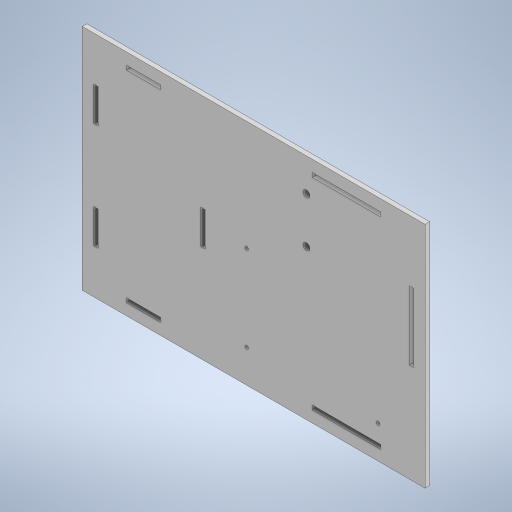
# Autodesk Inventor part: onderstuk_8AUG
Saved by Autodesk Inventor 2023.4 (Build 274418000, 418)
## iProperties
Created: 2024-07-29
Part Number: onderstuk_8AUG
Material: Generic
Document SubType Name: Modeling
Designer: cthey
Density: 1 g/cm^3
Appearance: Default
Author: cthey
Autodesk Inventor part; units mm, degrees
ref_plane "YZ Plane" through (0, 0, 0) normal (1, 0, 0) x (0, 1, 0)
ref_plane "XZ Plane" through (0, 0, 0) normal (0, 1, 0) x (-1, 0, 0)
ref_plane "XY Plane" through (0, 0, 0) normal (0, 0, 1) x (1, 0, 0)
sketch "Sketch1" plane through (0, 0, 0) normal (0, 0, 1) x (1, 0, 0)
  line L0 (0, 0) -> (300, 0)
  line L1 (300, 0) -> (300, 200)
  line L2 (300, 200) -> (0, 200)
  line L3 (0, 200) -> (0, 0)
  line L4 (10, 10) -> (290, 10)
  line L5 (290, 10) -> (290, 190)
  line L6 (290, 190) -> (10, 190)
  line L7 (10, 190) -> (10, 10)
  line L8 (13.75, 13.75) -> (286.25, 13.75)
  line L9 (286.25, 13.75) -> (286.25, 186.25)
  line L10 (286.25, 186.25) -> (13.75, 186.25)
  line L11 (13.75, 186.25) -> (13.75, 13.75)
  line L12 (38.75, 190) -> (68.5, 190)
  line L13 (68.5, 190) -> (68.5, 186.25)
  line L14 (68.5, 186.25) -> (38.75, 186.25)
  line L15 (38.75, 186.25) -> (38.75, 190)
  line L16 (10, 161.25) -> (13.75, 161.25)
  line L17 (13.75, 161.25) -> (13.75, 131.5)
  line L18 (13.75, 131.5) -> (10, 131.5)
  line L19 (10, 131.5) -> (10, 161.25)
  line L20 (0, 0) -> (150, 0)
  line L21 (150, 0) -> (150, 100)
  line L22 (150, 100) -> (0, 100)
  line L23 (0, 100) -> (0, 0)
  line L24 (38.75, 10) -> (68.5, 10)
  line L25 (68.5, 10) -> (68.5, 13.75)
  line L26 (68.5, 13.75) -> (38.75, 13.75)
  line L27 (38.75, 13.75) -> (38.75, 10)
  line L28 (10, 38.75) -> (13.75, 38.75)
  line L29 (13.75, 38.75) -> (13.75, 68.5)
  line L30 (13.75, 68.5) -> (10, 68.5)
  line L31 (10, 68.5) -> (10, 38.75)
  line L32 (150, 200) -> (150, 100)
  line L33 (300, 200) -> (300, 0)
  line L34 (261.25, 190) -> (231.5, 190)
  line L35 (231.5, 190) -> (231.5, 186.25)
  line L36 (231.5, 186.25) -> (261.25, 186.25)
  line L37 (261.25, 186.25) -> (261.25, 190)
  line L38 (290, 161.25) -> (286.25, 161.25)
  line L39 (286.25, 161.25) -> (286.25, 131.5)
  line L40 (286.25, 131.5) -> (290, 131.5)
  line L41 (290, 131.5) -> (290, 161.25)
  line L42 (300, 100) -> (300, 0)
  line L43 (261.25, 13.75) -> (261.25, 10)
  line L44 (231.5, 10) -> (231.5, 13.75)
  line L45 (231.5, 13.75) -> (261.25, 13.75)
  line L46 (261.25, 10) -> (231.5, 10)
  line L47 (286.25, 68.5) -> (290, 68.5)
  line L48 (290, 38.75) -> (286.25, 38.75)
  line L49 (290, 68.5) -> (290, 38.75)
  line L50 (286.25, 38.75) -> (286.25, 68.5)
  point P0 (13.75, 161.25)
  point P1 (10, 131.5)
  point P2 (10, 68.5)
  point P3 (13.75, 68.5)
  point P4 (13.75, 38.75)
  point P5 (10, 38.75)
  point P6 (68.5, 13.75)
  point P7 (68.5, 10)
  point P8 (38.75, 10)
  point P9 (38.75, 13.75)
  point P10 (231.5, 186.25)
  point P11 (231.5, 190)
  point P12 (261.25, 190)
  point P13 (261.25, 186.25)
  point P14 (286.25, 131.5)
  point P15 (286.25, 161.25)
  point P16 (290, 161.25)
  point P17 (261.25, 13.75)
  point P18 (261.25, 10)
  point P19 (231.5, 10)
  point P20 (231.5, 13.75)
  point P21 (286.25, 68.5)
  point P22 (286.25, 38.75)
  point P23 (68.5, 190)
  dimension "d0" = 300
  dimension "d1" = 200
  dimension "d2" = 280
  dimension "d3" = 180
  dimension "d4" = 10
  dimension "d5" = 10
  dimension "d6" = 3.75
  dimension "d7" = 3.75
  dimension "d8" = 3.75
  dimension "d9" = 3.75
  dimension "d10" = 25
  dimension "d11" = 29.75
  dimension "d12" = 29.75
  dimension "d13" = 25
  dimension "d14" = 100
  dimension "d15" = 150
  constraints: 102 end point, 26 symmetric about line, 12 parallel, 6 horizontal, 6 perpendicular, 4 point on line
  measures "d0" distance of L1.end L2.end
  measures "d1" distance of L0.end L1.end
  measures "d2" distance of L5.end L6.end
  measures "d3" distance of L6.end L4.start
  measures "d4" distance between parallel lines of L3 L7
  measures "d5" distance between parallel lines of L2 L6
  measures "d6" distance between parallel lines of L5 L9
  measures "d7" distance between parallel lines of L6 L10
  measures "d8" distance between parallel lines of L7 L11
  measures "d9" distance between parallel lines of L4 L8
  measures "d10" distance between parallel lines of L11 L15
  measures "d11" distance between parallel lines of L13 L15
  measures "d12" distance between parallel lines of L18 L16
  measures "d13" distance between parallel lines of L10 L16
  measures "d14" distance of L20.end L21.end
  measures "d15" distance of L21.end L22.end
extrude "Extrusion1" add sketch "Sketch1" along normal blind 4 contours L3 L22 L7 L4 L21 L0 | L21 L4 L5 L6 L32 L2 L1 L0 | L3 L2 L32 L6 L7 L22 | L21 L8 L44 L4 | L4 L25 L8 L21 | L22 L11 L30 L7 | L7 L18 L11 L22 | L21 L32 L10 L9 L8 | L8 L11 L22 L21 | L11 L10 L32 L22 | L4 L7 L28 L11 L8 L27 | L43 L8 L9 L48 L5 L4 | L32 L10 L13 L6 | L6 L35 L10 L32 | L7 L6 L15 L10 L11 L16 | L6 L5 L38 L9 L10 L37 | L47 L9 L40 L5
sketch "Sketch5" plane through (0, 0, 4) normal (0, 0, 1) x (1, 0, 0)
  line L0 (103.75, 114.875) -> (107.5, 114.875)
  line L1 (107.5, 114.875) -> (107.5, 85.125)
  line L2 (107.5, 85.125) -> (103.75, 85.125)
  line L3 (103.75, 85.125) -> (103.75, 114.875)
  line L4 (13.75, 68.5) -> (13.75, 38.75) projected
  line L5 (0, 0) -> (300, 0) projected
  point P0 (107.5, 100)
  dimension "d53" = 3.75
  dimension "d54" = 29.75
  dimension "d55" = 90
  dimension "d56" = 100
  constraints: 8 end point, 2 parallel, 1 horizontal, 1 midpoint, 1 perpendicular
  measures "d53" distance between parallel lines of L1 L3
  measures "d54" distance of L0.end L1.end
  measures "d55" distance between parallel lines of L4 L3
  measures "d56" distance from line of L5 point (107.5, 100)
extrude "Extrusion5" cut sketch "Sketch5" against normal through all
sketch "Sketch6" plane through (0, 0, 0) normal (0, 0, -1) x (-1, 0, 0)
  circle A0 centre (-258.8334, 28.75) radius 1.5
  circle A1 centre (-143.8334, 28.75) radius 1.5
  circle A2 centre (-143.8334, 103.75) radius 1.5
  line L0 (-300, 0) -> (-300, 200) projected
  line L1 (-231.5, 13.75) -> (-261.25, 13.75) projected
  circle A3 centre (-196.25, 171.25) radius 3
  circle A4 centre (-196.25, 131.25) radius 3
  line L2 (-286.25, 131.5) -> (-286.25, 161.25) projected
  line L3 (-261.25, 186.25) -> (-231.5, 186.25) projected
  point P0 (0, 0)
  dimension "d59" = 41.1666
  dimension "d60" = 115
  dimension "d61" = 75
  dimension "d62" = 0
  dimension "d63" = 3
  dimension "d64" = 3
  dimension "d65" = 3
  dimension "d66" = 15
  dimension "d67" = 15
  dimension "d70" = 40
  dimension "d71" = 6
  dimension "d72" = 6
  dimension "d73" = 90
  dimension "d74" = 90
  dimension "d75" = 15
  constraints: 5 centre point
  measures "d59" distance from line of A0.centre L0
  measures "d60" distance of A1.centre A0.centre
  measures "d61" distance of A1.centre A2.centre
  measures "d62" horizontal distance of A1.centre A2.centre
  measures "d63" diameter of A2
  measures "d64" diameter of A1
  measures "d65" diameter of A0
  measures "d66" distance from line of L1 A0.centre
  measures "d67" distance from line of L1 A1.centre
  measures "d70" distance of A4.centre A3.centre
  measures "d71" diameter of A3
  measures "d72" diameter of A4
  measures "d73" distance from line of L2 A3.centre
  measures "d74" distance from line of L2 A4.centre
  measures "d75" distance from line of L3 A3.centre
extrude "Extrusion6" cut sketch "Sketch6" against normal through all
sketch "Sketch7" plane through (0, 0, 0) normal (0, 0, -1) x (-1, 0, 0)
  line L0 (-290, 146.5) -> (-286.25, 146.5)
  line L1 (-286.25, 146.5) -> (-286.25, 86.5)
  line L2 (-286.25, 86.5) -> (-290, 86.5)
  line L3 (-290, 86.5) -> (-290, 146.5)
  line L4 (-290, 161.25) -> (-290, 131.5) projected
  line L5 (-286.25, 131.5) -> (-286.25, 161.25) projected
  line L6 (-290, 131.5) -> (-286.25, 131.5) projected
  line L7 (-290, 68.5) -> (-290, 38.75) projected
  line L8 (-286.25, 38.75) -> (-286.25, 68.5) projected
  line L9 (-290, 68.5) -> (-286.25, 68.5)
  line L10 (-286.25, 68.5) -> (-286.25, 38.75)
  line L11 (-286.25, 38.75) -> (-290, 38.75)
  line L12 (-290, 38.75) -> (-290, 68.5)
  line L13 (-290, 161.25) -> (-290, 131.5) projected
  line L14 (-290, 161.25) -> (-286.25, 161.25)
  line L15 (-286.25, 161.25) -> (-286.25, 146.5)
  line L16 (-286.25, 146.5) -> (-290, 146.5)
  line L17 (-290, 146.5) -> (-290, 161.25)
  point P0 (0, 0)
  dimension "d79" = 0
  dimension "d80" = 0
  dimension "d81" = 15
  dimension "d82" = 60
  constraints: 24 end point, 6 parallel, 3 horizontal, 3 perpendicular
  measures "d79" distance between parallel lines of L4 L3
  measures "d80" distance between parallel lines of L5 L1
  measures "d81" distance between parallel lines of L6 L0
  measures "d82" distance between parallel lines of L0 L2
extrude "Extrusion7" add sketch "Sketch7" against normal blind 4 contours L4 L14 L5 L0 | L9 L8 L11 L7
extrude "Extrusion8" cut sketch "Sketch7" against normal through all contours L0 L1 L6 L3 | L6 L1 L2 L3
sketch "Sketch8" plane through (0, 0, 0) normal (0, 0, -1) x (-1, 0, 0)
  line L0 (-261.25, 190) -> (-261.25, 186.25) projected
  line L1 (-261.25, 190) -> (-201.25, 190)
  line L2 (-201.25, 190) -> (-201.25, 186.25)
  line L3 (-201.25, 186.25) -> (-261.25, 186.25)
  line L4 (-261.25, 186.25) -> (-261.25, 190)
  line L5 (-261.25, 13.75) -> (-261.25, 10) projected
  line L6 (-261.25, 13.75) -> (-201.25, 13.75)
  line L7 (-201.25, 13.75) -> (-201.25, 10)
  line L8 (-201.25, 10) -> (-261.25, 10)
  line L9 (-261.25, 10) -> (-261.25, 13.75)
  point P0 (0, 0)
  dimension "d87" = 60
  dimension "d88" = 3.75
  dimension "d89" = 3.75
  constraints: 16 end point, 4 parallel, 2 horizontal, 2 perpendicular, 1 point on line
  measures "d87" distance of L2.end L3.end
  measures "d88" distance of L1.end L2.end
  measures "d89" distance between parallel lines of L6 L8
extrude "Extrusion9" cut sketch "Sketch8" against normal through all
body "Solid1"
